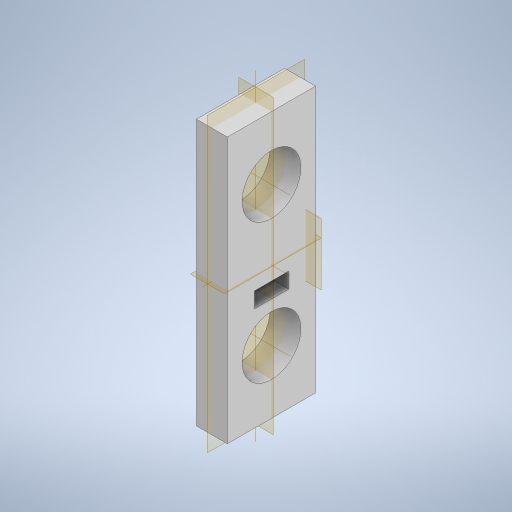
# Autodesk Inventor part: E-Axis v2.0
Saved by Autodesk Inventor 2023 (Build 270158000, 158)
## iProperties
Created: 2023-07-26
Part Number: E-Axis v2.0
Material: Generic
Document SubType Name: Modeling
Designer: Parker
Density: 1 g/cm^3
Appearance: Default
Author: Parker
Autodesk Inventor part; units mm, degrees
ref_plane "UpperRodPlane" through (0, 22.5, 0) normal (0, 1, 0) x (-1, 0, 0)
ref_plane "LowerRodPlane" through (0, -22.5, 0) normal (0, 1, 0) x (-1, 0, 0)
ref_plane "RearClearancePlane" through (0, 0, -11) normal (0, 0, 1) x (1, 0, 0)
sketch "Sketch1" plane through (0, 0, 0) normal (1, 0, 0) x (0, 1, 0)
  circle A0 centre (22.5, 0) radius 9.5
  circle A1 centre (-22.5, 0) radius 9.5
  line L0 (-4.5, 5.5) -> (-9.5, 5.5)
  line L1 (-9.5, 5.5) -> (-9.5, -5.5)
  line L2 (-9.5, -5.5) -> (-4.5, -5.5)
  line L3 (-4.5, -5.5) -> (-4.5, 5.5)
  line L4 (-4.5, 5.5) -> (-9.5, -5.5) construction
  line L5 (-9.5, 5.5) -> (-4.5, -5.5) construction
  line L6 (42.8516, -14.2259) -> (-42.8516, -14.2259)
  line L7 (-42.8516, -14.2259) -> (-42.8516, 14.2259)
  line L8 (-42.8516, 14.2259) -> (42.8516, 14.2259)
  line L9 (42.8516, 14.2259) -> (42.8516, -14.2259)
  line L10 (42.8516, -14.2259) -> (-42.8516, 14.2259) construction
  line L11 (-42.8516, -14.2259) -> (42.8516, 14.2259) construction
  point P0 (0, 0)
  point P1 (-7, 0)
  dimension "d3" = 19
  dimension "d4" = 19
  dimension "d5" = 11
  dimension "d6" = 13
  dimension "d7" = 27
  constraints: 24 end point, 4 midpoint, 4 parallel, 2 centre point, 2 coincident, 2 horizontal, 2 perpendicular, 1 horizontal alignment
  measures "d3" diameter of A0
  measures "d4" diameter of A1
  measures "d5" distance of L1.end L0.end
  measures "d6" distance from line of L1 point (-22.5, 0)
  measures "d7" distance from line of L3 A0.centre
extrude "Extrusion1" add sketch "Sketch1" along normal mid plane 10
body "Solid1"
